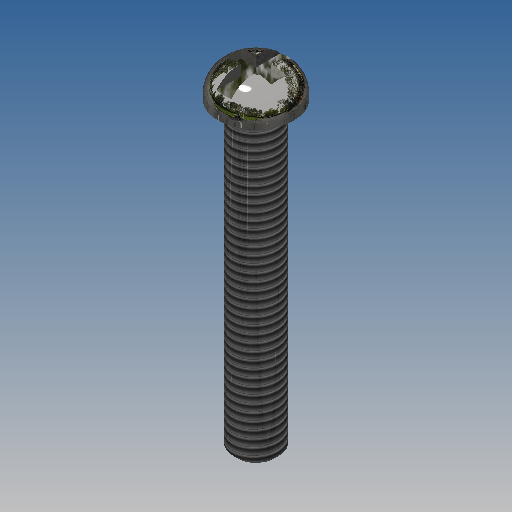
# Autodesk Inventor part: M3x10 Screw Nylon
Saved by Autodesk Inventor 2017 (Build 210142000, 142)
## iProperties
Created: 2016-02-18
Part Number: M3x10 Screw Nylon
Material: Steel
Document SubType Name: Modeling
Designer: 23902
Density: 7.85 g/cm^3
Appearance: Plate
Mass: 0.113453 g
Surface Area: 1.50413 cm^2
Volume: 0.101298 cm^3
Author: 23902
Autodesk Inventor part; units mm, degrees
ref_plane "YZ Plane" through (0, 0, 0) normal (1, 0, 0) x (0, 1, 0)
ref_plane "XZ Plane" through (0, 0, 0) normal (0, 1, 0) x (-1, 0, 0)
ref_plane "XY Plane" through (0, 0, 0) normal (0, 0, 1) x (1, 0, 0)
sketch "Sketch1" plane through (0, 0, 0) normal (0, 1, 0) x (-1, 0, 0)
  circle A0 centre (0, 0) radius 1.5
  dimension "d0" = 3
  constraints: 1 centre point, 1 coincident
  measures "d0" diameter of A0
extrude "Extrusion1" add sketch "Sketch1" along normal blind 20
sketch "Sketch2" plane through (0, 20, 0) normal (0, 1, 0) x (1, 0, 0)
  circle A0 centre (0, 0) radius 2.5
  dimension "d3" = 5
  constraints: 1 centre point, 1 coincident
  measures "d3" diameter of A0
extrude "Extrusion2" add sketch "Sketch2" along normal blind 2
fillet "Fillet1" radius 1.7 1 edges at (-2.5, 22, 0)
chamfer "Chamfer1" distance 0.3 angle 45 1 edges at (1.5, 0, 0)
thread "Thread1" size "M3x0.5" class "6g" standard "ANSI Metric M Profile" full length
sketch "Sketch3" plane through (0, 22, 0) normal (0, 1, 0) x (1, 0, 0)
  line L0 (0.5, -2.5) -> (0.5, 2.5)
  line L1 (0.5, 2.5) -> (-0.5, 2.5)
  line L2 (-0.5, 2.5) -> (-0.5, -2.5)
  line L3 (-0.5, -2.5) -> (0.5, -2.5)
  line L4 (0.5, -2.5) -> (-0.5, 2.5) construction
  line L5 (0.5, 2.5) -> (-0.5, -2.5) construction
  line L6 (1.5, -0.5) -> (-1.5, -0.5)
  line L7 (-1.5, -0.5) -> (-1.5, 0.5)
  line L8 (-1.5, 0.5) -> (1.5, 0.5)
  line L9 (1.5, 0.5) -> (1.5, -0.5)
  circle A0 centre (0, 0) radius 2.5 projected
  line L10 (1.5, -0.5) -> (-1.5, 0.5) construction
  line L11 (-1.5, -0.5) -> (1.5, 0.5) construction
  dimension "d12" = 1
  dimension "d13" = 3
  dimension "d14" = 1
  constraints: 24 end point, 5 parallel, 4 midpoint, 2 perpendicular, 1 vertical
  measures "d12" distance of L1.end L0.end
  measures "d13" distance of L6.start L6.end
  measures "d14" distance of L6.end L7.end
extrude "Extrusion3" cut sketch "Sketch3" against normal blind 0.7 contours L3 A0 L0 | A0 L2 L6 L0 | L3 L2 A0 | L6 L2 L8 L0 | L0 L8 L9 L6 | L8 L2 A0 L0 | L6 L7 L8 L2 | A0 L1 L0 | L2 L1 A0
body "Solid1"
